Autodesk Fusion 360 part; units mm, degrees
note: some values were not read from the file. Chosen so that the rebuilt part matches the saved one: a direction; where a step ends. Set by a fixed rule: which sketch regions a step uses.
(part 2 of 2)
equation "d172 = ( d174 - d169 ) / 2"
equation "d175 = d174"
equation "d176 = d167"
equation "d178 = d160"
equation "d179 = distance_screws"
equation "d180 = screws_dia - kerf"
equation "d181 = d163"
equation "d185 = height_screws + thickness"
equation "d188 = d160"
equation "d189 = distance_screws"
equation "d190 = screws_dia - kerf"
equation "d191 = screws_dia - kerf"
equation "d195 = d188"
equation "distance_screws_eggslider = 34 mm"
equation "d286 = 3.5 mm - kerf"
equation "d287 = d286"
equation "d288 = d287"
equation "d289 = d288"
equation "d290 = distance_screws_eggslider"
equation "d291 = distance_screws_eggslider"
equation "d292 = distance_screws_eggslider"
equation "distance_screws_eggslider_axis = 35.2 mm"
equation "d321 = -thickness"
equation "d323 = screws_dia - kerf"
equation "d324 = screws_dia - kerf"
equation "d325 = distance_screws"
equation "d326 = d327"
equation "d327 = height_screws + thickness"
equation "d328 = ( d329 - d325 ) / 2"
equation "d365 = ( d364 - d179 ) / 2"
equation "d366 = d185"
equation "d368 = ( d367 - d189 ) / 2"
equation "d369 = d195"
equation "d455 = width_mounts / 3 + kerf"
equation "d456 = ( d16 - d455 ) / 2"
equation "d457 = d455"
equation "d458 = d456"
equation "d459 = d457"
equation "d460 = d456"
equation "d461 = d456"
equation "d462 = d455"
equation "d463 = d461"
equation "d464 = d462"
equation "d465 = thickness - 0.5 * kerf"
equation "d466 = width_mounts / 3 - kerf"
equation "d467 = ( d166 - d466 ) / 2"
equation "d468 = thickness - 0.5 * kerf"
equation "d469 = ( d175 - d470 ) / 2"
equation "d470 = width_mounts / 3 - kerf"
equation "d471 = thickness - 0.5 * kerf"
equation "d472 = ( d364 - d473 ) / 2"
equation "d473 = width_mounts / 3 - kerf"
equation "d474 = width_mounts / 3 - kerf"
equation "d475 = thickness - 0.5 * kerf"
equation "d476 = ( d367 - d474 ) / 2"
equation "d477 = thickness - 0.5 * kerf"
equation "d478 = ( d329 - d479 ) / 2"
equation "d479 = width_mounts / 3 - kerf"
equation "d480 = distance_screws_eggslider_axis"
equation "d481 = d480"
equation "d482 = d481"
equation "d483 = d482"
equation "d484 = d480"
equation "d485 = d481"
equation "d486 = d482"
equation "d487 = d483"
equation "d492 = screws_dia - kerf"
equation "d493 = d492"
equation "d494 = d492"
equation "d495 = d492"
equation "d496 = d492"
equation "d497 = d492"
equation "d498 = d492"
equation "d499 = d492"
equation "d500 = height_screws"
equation "d501 = d500"
equation "d502 = height_screws"
equation "d503 = d502"
equation "d504 = d503"
equation "d505 = d503"
equation "d506 = d504"
equation "d507 = d504"
equation "d508 = distance_screws / 2"
equation "d509 = distance_screws / 2"
equation "d510 = distance_screws / 2"
equation "d511 = distance_screws / 2"
equation "d512 = distance_screws / 2"
equation "d513 = distance_screws / 2"
equation "d514 = distance_screws / 2"
equation "d515 = distance_screws / 2"
equation "d520 = d88"
equation "d523 = thickness"
equation "d525 = thickness + height_screws"
equation "d526 = d525"
equation "d527 = 3.5 mm - kerf"
equation "d528 = d527"
equation "d529 = distance_screws"
equation "d531 = ( d530 - d529 ) / 2"
equation "d532 = width_mounts / 3 - kerf"
equation "d533 = thickness - 0.5 * kerf"
equation "d534 = ( d530 - d532 ) / 2"
